saddle_coupon (Autodesk Fusion 360 design; units mm, degrees)
part number: 2026-09-02-15-56-22-744
Autodesk Fusion 360 part; units mm, degrees
sketch "Coupon chord" plane through (0, 0, 0) normal (0, 1, 0) x (1, 0, 0)
  line L0 (70, -76) -> (150, -76)
  line L1 (150, -76) -> (150, -90)
  line L2 (150, -90) -> (70, -90)
  line L3 (70, -90) -> (70, -76)
  dimension "d52" = 70
  dimension "d53" = 76
  dimension "d55" = 90
  constraint horizontal L0
  constraint horizontal L2
  constraint vertical L1
  constraint vertical L3
  measures "d52" horizontal distance of origin L0.start
  measures "d53" vertical distance of origin L0.start
  measures "d55" vertical distance of origin L1.end
extrude "Coupon chord (1)" add sketch "Coupon chord" along normal mid plane 8
sketch "Saddle boss x=70" plane through (0, 0, 0) normal (0, 1, 0) x (1, 0, 0)
  circle A0 centre (70, -90) radius 22.7
  dimension "d58" = 70
  dimension "d59" = 90
  dimension "d60" = 45.4
  measures "d58" horizontal distance of origin A0.centre
  measures "d59" vertical distance of origin A0.centre
  measures "d60" diameter of A0
extrude "Saddle boss x=70 (1)" add sketch "Saddle boss x=70" along normal mid plane 8
sketch "Saddle boss x=150" plane through (0, 0, 0) normal (0, 1, 0) x (1, 0, 0)
  circle A0 centre (150, -90) radius 22.7
  dimension "d64" = 90
  dimension "d65" = 45.4
  measures "d64" vertical distance of origin A0.centre
  measures "d65" diameter of A0
extrude "Saddle boss x=150 (1)" add sketch "Saddle boss x=150" along normal mid plane 8
sketch "Rod pocket x=70" plane through (0, 0, 0) normal (0, 1, 0) x (1, 0, 0)
  circle A0 centre (70, -90) radius 17.1
  dimension "d68" = 70
  dimension "d69" = 90
  dimension "d70" = 34.2
  measures "d68" horizontal distance of origin A0.centre
  measures "d69" vertical distance of origin A0.centre
  measures "d70" diameter of A0
extrude "Rod pocket x=70 (1)" cut sketch "Rod pocket x=70" along normal mid plane 18
sketch "Drop-in opening x=70" plane through (0, 0, 0) normal (0, 1, 0) x (1, 0, 0)
  line L0 (52.9, -90) -> (87.1, -90)
  line L1 (87.1, -90) -> (87.1, -117.7)
  line L2 (87.1, -117.7) -> (52.9, -117.7)
  line L3 (52.9, -117.7) -> (52.9, -90)
  dimension "d73" = 52.9
  dimension "d74" = 90
  dimension "d75" = 87.1
  dimension "d76" = 117.7
  constraint horizontal L0
  constraint horizontal L2
  constraint vertical L1
  constraint vertical L3
  measures "d73" horizontal distance of origin L0.start
  measures "d74" vertical distance of origin L0.start
  measures "d75" horizontal distance of origin L1.end
  measures "d76" vertical distance of origin L1.end
extrude "Drop-in opening x=70 (1)" cut sketch "Drop-in opening x=70" along normal mid plane 18
sketch "Rod pocket x=150" plane through (0, 0, 0) normal (0, 1, 0) x (1, 0, 0)
  circle A0 centre (150, -90) radius 17.1
  dimension "d80" = 90
  dimension "d81" = 34.2
  measures "d80" vertical distance of origin A0.centre
  measures "d81" diameter of A0
extrude "Rod pocket x=150 (1)" cut sketch "Rod pocket x=150" along normal mid plane 18
sketch "Drop-in opening x=150" plane through (0, 0, 0) normal (0, 1, 0) x (1, 0, 0)
  line L0 (132.9, -90) -> (167.1, -90)
  line L1 (167.1, -90) -> (167.1, -117.7)
  line L2 (167.1, -117.7) -> (132.9, -117.7)
  line L3 (132.9, -117.7) -> (132.9, -90)
  dimension "d84" = 132.9
  dimension "d85" = 90
  dimension "d86" = 167.1
  dimension "d87" = 117.7
  constraint horizontal L0
  constraint horizontal L2
  constraint vertical L1
  constraint vertical L3
  measures "d84" horizontal distance of origin L0.start
  measures "d85" vertical distance of origin L0.start
  measures "d86" horizontal distance of origin L1.end
  measures "d87" vertical distance of origin L1.end
extrude "Drop-in opening x=150 (1)" cut sketch "Drop-in opening x=150" along normal mid plane 18
equation "couponWidth = 8.0 mm" comment "coupon slice width"
equation "plateHeight = 90.0 mm" comment "rod height, as the bracket"
equation "rodOuterDiameter = 33.4 mm" comment "1 inch sch 40 PVC"
equation "saddleClearance = 0.8 mm" comment "diametral pocket clearance"
equation "saddleWall = 6.0 mm" comment "wall around the rod pocket"
equation "rearRodStandoff = 70.0 mm" comment "rear rod, from the upright"
equation "rodSpacing = 80.0 mm" comment "rod centres, front minus rear"
equation "memberWidth = 14.0 mm" comment "chord depth joining the saddles"
equation "d52 = rearRodStandoff"
equation "d53 = plateHeight - memberWidth"
equation "d54 = ( rearRodStandoff + rodSpacing )"
equation "d55 = plateHeight"
equation "d56 = couponWidth"
equation "d58 = rearRodStandoff"
equation "d59 = plateHeight"
equation "d60 = rodOuterDiameter + 2 * saddleWall"
equation "d61 = couponWidth"
equation "d63 = ( rearRodStandoff + rodSpacing )"
equation "d64 = plateHeight"
equation "d65 = rodOuterDiameter + 2 * saddleWall"
equation "d66 = couponWidth"
equation "d68 = rearRodStandoff"
equation "d69 = plateHeight"
equation "d70 = rodOuterDiameter + saddleClearance"
equation "d71 = couponWidth + 10 mm"
equation "d73 = rearRodStandoff - ( rodOuterDiameter + saddleClearance ) / 2"
equation "d74 = plateHeight"
equation "d75 = rearRodStandoff + ( rodOuterDiameter + saddleClearance ) / 2"
equation "d76 = plateHeight + ( rodOuterDiameter + 2 * saddleWall ) / 2 + 5 mm"
equation "d77 = couponWidth + 10 mm"
equation "d79 = ( rearRodStandoff + rodSpacing )"
equation "d80 = plateHeight"
equation "d81 = rodOuterDiameter + saddleClearance"
equation "d82 = couponWidth + 10 mm"
equation "d84 = ( rearRodStandoff + rodSpacing ) - ( rodOuterDiameter + saddleClearance ) / 2"
equation "d85 = plateHeight"
equation "d86 = ( rearRodStandoff + rodSpacing ) + ( rodOuterDiameter + saddleClearance ) / 2"
equation "d87 = plateHeight + ( rodOuterDiameter + 2 * saddleWall ) / 2 + 5 mm"
equation "d88 = couponWidth + 10 mm"
named bodies: "saddle_coupon"
